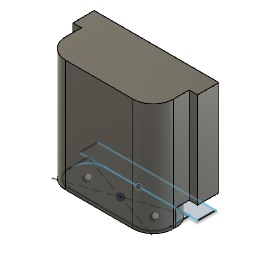
Mid Layer - Left No Macro Rev 2 v3 (Autodesk Fusion 360 archive; units mm, degrees)
design "USB C Punch - 0.3mm Expanded"
Autodesk Fusion 360 part; units mm, degrees
sketch "Sketch1" plane through (0, 0, 0) normal (0, 1, 0) x (1, 0, 0)
  line L0 (4.5, 1.6) -> (-4.5, 1.6)
  line L1 (-4.5, 0.1) -> (-4.5, -0.1)
  line L2 (-3, -1.6) -> (3, -1.6)
  line L3 (4.5, -0.1) -> (4.5, 0.1)
  line L4 (4.5, 1.6) -> (-4.5, -1.6) construction
  line L5 (-4.5, 1.6) -> (4.5, -1.6) construction
  arc A0 (-4.5, -0.1) -> (-3, -1.6) centre (-3, -0.1) ccw
  arc A1 (3, -1.6) -> (4.5, -0.1) centre (3, -0.1) ccw
  line L6 (3, 1.6) -> (-3, 1.6)
  arc A2 (-3, 1.6) -> (-4.5, 0.1) centre (-3, 0.1) ccw
  arc A3 (4.5, 0.1) -> (3, 1.6) centre (3, 0.1) ccw
  line L7 (4.5, 1.6) -> (4.5, 0)
  line L8 (-4.5, 1.6) -> (-4.5, 0)
  line L9 (-5.25, 3.2) -> (5.25, 3.2)
  line L10 (5.25, 3.2) -> (5.25, 1.6)
  line L11 (5.25, 1.6) -> (-5.25, 1.6)
  line L12 (-5.25, 1.6) -> (-5.25, 3.2)
  point P0 (0, 1.6)
  point P1 (0, 1.6)
  dimension "d5" = 9
  dimension "d6" = 3.2
  dimension "d8" = 1.5
  dimension "d11" = 1.5
  dimension "d12" = 10.5
  dimension "d13" = 1.6
  constraint horizontal L0
  constraint perpendicular L0 L1
  constraint parallel L0 L2
  constraint parallel L1 L3
  constraint coincident L4 origin
  constraint coincident L5 origin
  constraint coincident L4.end L1
  constraint coincident L4.end L2
  constraint tangent L1 A0
  constraint tangent L2 A0
  constraint coincident L5.end L3
  constraint coincident L5.end L2
  constraint tangent L3 A1
  constraint tangent L2 A1
  constraint equal A0 A1
  constraint horizontal L6
  constraint coincident L6 P1
  constraint coincident L0.end L1
  constraint tangent L1 A2
  constraint tangent L6 A2
  constraint coincident L0.start L3
  constraint tangent L3 A3
  constraint tangent L6 A3
  constraint equal A2 A3
  constraint midpoint L3 L7.end
  constraint midpoint L1 L8.end
  constraint horizontal L9
  constraint vertical L10
  constraint horizontal L11
  constraint vertical L12
  constraint midpoint L11 P1
  constraint midpoint L6 P1
  measures "d5" distance of L4.end L5.end
  measures "d6" distance of L0.end L4.end
  measures "d8" radius of A0
  measures "d11" radius of A2
  measures "d12" distance of L9.start L9.end
  measures "d13" distance of L9.start L11.end
extrude "Extrude1" add sketch "Sketch1" along normal blind 10 contours L0 L1 L2 L3 A0 A1 L6 A2 A3 L7 L8 L11
extrude "Extrude2" add sketch "Sketch1" along normal blind 8.5 from surface at 1.5 contours L0 A3 L7 L11 | L0 L6 L9 L10 L11 L12 | L0 A2 L8 L11
move_face "OffsetFaces1" offset 0.3 12 faces at (4.4983, 6.6667, 0.1714) (-1, 3.3333, 1.6) (-3.0714, 6.6667, 1.5983) (-4.5, 7.1667, -0.5333) (-4.75, 4.3333, -1.6) (-5.25, 4.3333, -2.1333) (4.5, 7.1667, -0.5333) (3.0714, 1, -1.5983) (1, 0.5, -1.6) (-4.3926, 1, -0.6575) (5, 4.3333, -1.6) (5.25, 4.3333, -2.6667)
equation "usb_c_width = 9 mm"
equation "usb_c_height = 3.2 mm"
equation "pcb_thickness = 1.6 mm"
equation "pcb_width = 10.5 mm"
equation "d5 = usb_c_width"
equation "d6 = usb_c_height"
equation "usb_c_fillet = 1.5 mm"
equation "d8 = usb_c_fillet"
equation "d11 = usb_c_fillet"
equation "d12 = pcb_width"
equation "d13 = pcb_thickness"
